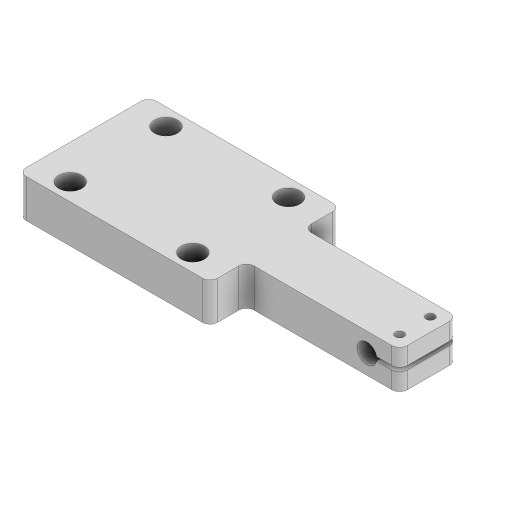
# Autodesk Inventor part: Puller
Saved by Autodesk Inventor 2023 (Build 270158000, 158)
## iProperties
Created: 2026-05-19
Part Number: Puller
Material: Generic
Document SubType Name: Modeling
Designer: ferrerx
Density: 1 g/cm^3
Appearance: Default
Author: ferrerx
Autodesk Inventor part; units mm, degrees
ref_plane "YZ Plane" through (0, 0, 0) normal (1, 0, 0) x (0, 1, 0)
ref_plane "XZ Plane" through (0, 0, 0) normal (0, 1, 0) x (-1, 0, 0)
ref_plane "XY Plane" through (0, 0, 0) normal (0, 0, 1) x (1, 0, 0)
sketch "Sketch1" plane through (0, 0, 0) normal (0, 1, 0) x (-1, 0, 0)
  line L0 (-16, 12.5) -> (16, 12.5) construction
  line L1 (16, 12.5) -> (16, -12.5) construction
  line L2 (16, -12.5) -> (-16, -12.5) construction
  line L3 (-16, -12.5) -> (-16, 12.5) construction
  line L4 (-16, 12.5) -> (16, -12.5) construction
  line L5 (16, 12.5) -> (-16, -12.5) construction
  circle A0 centre (16, 12.5) radius 1.65
  circle A1 centre (16, -12.5) radius 1.65
  circle A2 centre (-16, -12.5) radius 1.65
  circle A3 centre (-16, 12.5) radius 1.65
  line L6 (-25, 17) -> (25, 17)
  line L7 (25, 17) -> (25, -17)
  line L8 (25, -17) -> (-25, -17)
  line L9 (-25, -17) -> (-25, 17)
  line L10 (-25, 17) -> (25, -17) construction
  line L11 (25, 17) -> (-25, -17) construction
  point P0 (0, 0)
  dimension "d0" = 32
  dimension "d1" = 25
  dimension "d2" = 3.3
  dimension "d3" = 3.3
  dimension "d4" = 3.3
  dimension "d5" = 3.3
  dimension "d6" = 50
  dimension "d7" = 34
  constraints: 24 end point, 4 centre point, 4 coincident, 4 midpoint, 4 parallel, 2 horizontal, 2 perpendicular
  measures "d0" distance of L1.end L2.end
  measures "d1" distance of L0.end L1.end
  measures "d2" diameter of A0
  measures "d3" diameter of A1
  measures "d4" diameter of A2
  measures "d5" diameter of A3
  measures "d6" distance of L7.end L8.end
  measures "d7" distance of L6.end L7.end
extrude "Extrusion1" add sketch "Sketch1" along normal blind 10
sketch "Sketch2" plane through (0, 10, 0) normal (0, 1, 0) x (1, 0, 0)
  line L0 (-24, -7.5) -> (-12, -7.5)
  line L1 (-12, -7.5) -> (-12, 7.5)
  line L2 (-12, 7.5) -> (-24, 7.5)
  line L3 (-24, 7.5) -> (-24, -7.5)
  line L4 (-24, -7.5) -> (-12, 7.5) construction
  line L5 (-12, -7.5) -> (-24, 7.5) construction
  circle A0 centre (-16, -12.5) radius 1.65 projected
  circle A1 centre (-16, -12.5) radius 3 construction
  point P0 (0, 0)
  point P1 (-18, 0)
  dimension "d10" = 18
  dimension "d11" = 15
  dimension "d12" = 6
  dimension "d13" = 12
  constraints: 12 end point, 2 midpoint, 2 parallel, 1 centre point, 1 coincident, 1 horizontal, 1 perpendicular
  measures "d10" distance of point (0, 0) point (-18, 0)
  measures "d11" distance of L2.end L0.start
  measures "d12" diameter of A1
  measures "d13" distance of L1.end L2.end
extrude "Extrusion2" [suppressed]
sketch "Sketch5" plane through (0, 0, 0) normal (0, 0, 1) x (1, 0, 0)
  line L0 (25, 10) -> (-25, 10) projected
  line L1 (-21.2587, 10) -> (-11, 10)
  line L2 (-11, 10) -> (-11, 19.7515)
  line L3 (-11, 19.7515) -> (-17.6064, 31.6553)
  line L4 (-17.6064, 31.6553) -> (-28.0988, 25.8321)
  line L5 (-28.0988, 25.8321) -> (-21.2587, 13.5072)
  line L6 (-21.2587, 13.5072) -> (-21.2587, 10)
  circle A0 centre (-18, 20) radius 2.6308
  line L7 (-25, 0) -> (-25, 10) projected
  point P0 (0, 0)
  dimension "d22" = 7
  dimension "d23" = 10
  dimension "d24" = 7
  dimension "d26" = 6
  dimension "d27" = 6
  dimension "d28" = 10
  constraints: 13 end point, 2 perpendicular, 2 point on line, 1 centre point, 1 parallel, 1 vertical
  measures "d22" distance from line of L7 A0.centre
  measures "d23" distance from line of L0 A0.centre
  measures "d24" distance from line of A0.centre L2
  measures "d26" distance from line of L5 A0.centre
  measures "d27" distance from line of L3 A0.centre
  measures "d28" distance from line of A0.centre L4
extrude "Extrusion4" [suppressed]
sketch "Sketch6" plane through (-17.6064, 27.6553, 6) normal (0.8744, 0.4853, 0) x (0, 0, -1)
  circle A0 centre (3, -3) radius 1.1
  line L0 (12, 0) -> (0, 0) projected
  line L1 (0, -13.6141) -> (0, 0) projected
  line L2 (6, 0) -> (6, -13.6141) construction
  line L3 (12, -13.6141) -> (0, -13.6141) projected
  circle A1 centre (9, -3) radius 1.1
  point P0 (6, -32.7246)
  dimension "d31" = 3
  dimension "d32" = 3
  dimension "d38" = 2.2
  constraints: 2 centre point, 2 end point, 2 midpoint, 1 symmetric about line, 1 other
  measures "d31" distance from line of L0 A0.centre
  measures "d32" distance from line of L1 A0.centre
  measures "d38" diameter of A0
extrude "Extrusion5" [suppressed]
sketch "Sketch7" plane through (0, 0, 6) normal (0, 0, 1) x (1, 0, 0)
  line L0 (-28.2228, 33.3896) -> (-18.3568, 15.6125)
  line L1 (-18.3568, 15.6125) -> (-17.4824, 16.0978)
  line L2 (-17.4824, 16.0978) -> (-27.3485, 33.8749)
  line L3 (-27.3485, 33.8749) -> (-28.2228, 33.3896)
  line L4 (-17.6064, 27.6553) -> (-28.0988, 21.8321) projected
  line L5 (-28.2228, 33.3896) -> (-17.4824, 16.0978) construction
  line L6 (-18.3568, 15.6125) -> (-27.3485, 33.8749) construction
  point P0 (0, 0)
  point P1 (-22.8526, 24.7437)
  dimension "d35" = 1
  constraints: 12 end point, 3 midpoint, 2 parallel, 2 perpendicular
  measures "d35" distance between parallel lines of L2 L0
extrude "Extrusion6" [suppressed]
sketch "Sketch8" plane through (-21.2587, 9.5072, -6) normal (-0.8744, -0.4853, 0) x (0, 0, 1)
  circle A0 centre (9, 11.0958) radius 1.1 projected
  circle A1 centre (9, 11.0958) radius 1.65
  circle A2 centre (3, 11.0958) radius 1.1 projected
  circle A3 centre (3, 11.0958) radius 1.65
  point P0 (6, -18.6288)
  dimension "d39" = 3.3
  dimension "d40" = 3.3
  constraints: 2 centre point, 2 coincident
  measures "d39" diameter of A3
  measures "d40" diameter of A1
extrude "Extrusion7" [suppressed]
fillet "Fillet1" [suppressed]
chamfer "Chamfer1" [suppressed]
sketch "Sketch9" plane through (0, 10, 0) normal (0, 1, 0) x (1, 0, 0)
  circle A0 centre (-16, 12.5) radius 1.65 projected
  circle A1 centre (-16, 12.5) radius 3
  circle A2 centre (16, 12.5) radius 1.65 projected
  circle A3 centre (16, 12.5) radius 3
  circle A4 centre (16, -12.5) radius 1.65 projected
  circle A5 centre (16, -12.5) radius 3
  circle A6 centre (-16, -12.5) radius 1.65 projected
  circle A7 centre (-16, -12.5) radius 3
  point P0 (0, 0)
  dimension "d47" = 6
  dimension "d48" = 6
  dimension "d49" = 6
  dimension "d50" = 6
  constraints: 4 centre point, 4 coincident
  measures "d47" diameter of A1
  measures "d48" diameter of A3
  measures "d49" diameter of A5
  measures "d50" diameter of A7
extrude "Extrusion8" cut sketch "Sketch9" against normal blind 4 contours A0 | A1 | A3 | A5 | A7
fillet "Fillet2" radius 2 4 edges at (25, 5, 17) (25, 5, -17) (-25, 5, 17) (-25, 5, -17)
sketch "Sketch11" plane through (0, 0, 0) normal (0, 0, 1) x (1, 0, 0)
  line L0 (25, 10) -> (-25, 10) projected
  line L1 (25, 10) -> (65, 10)
  line L2 (65, 10) -> (65, 0)
  line L3 (65, 0) -> (25, 0)
  line L4 (25, 0) -> (25, 10)
  point P0 (0, 0)
  dimension "d54" = 40
  dimension "d55" = 10
  constraints: 8 end point, 2 parallel, 1 horizontal, 1 perpendicular
  measures "d54" distance of L0.start L1.end
  measures "d55" distance of L1.end L2.end
extrude "Extrusion9" add sketch "Sketch11" along normal mid plane 15
sketch "Sketch12" plane through (0, 0, -7.5) normal (0, 0, -1) x (-1, 0, 0)
  line L0 (-65, 10) -> (-65, 0) projected
  line L1 (-65, 5) -> (-56.5, 5) construction
  circle A0 centre (-56.5, 5) radius 2.55
  line L2 (-67.1062, 5.5) -> (-57.7546, 5.5)
  line L3 (-57.7546, 5.5) -> (-57.7546, 4.5)
  line L4 (-57.7546, 4.5) -> (-67.1062, 4.5)
  line L5 (-67.1062, 4.5) -> (-67.1062, 5.5)
  line L6 (-67.1062, 5.5) -> (-57.7546, 4.5) construction
  line L7 (-57.7546, 5.5) -> (-67.1062, 4.5) construction
  point P0 (0, 0)
  point P1 (-62.4304, 5)
  point P2 (-59.0005, 4.5)
  point P3 (-59.0005, 5.5)
  dimension "d58" = 5.1
  dimension "d59" = 8.5
  dimension "d67" = 1
  constraints: 14 end point, 3 midpoint, 2 horizontal, 2 parallel, 1 centre point, 1 coincident, 1 perpendicular, 1 point on line
  measures "d58" diameter of A0
  measures "d59" distance of L1.start L1.end
  measures "d67" distance between parallel lines of L2 L4
extrude "Extrusion10" cut sketch "Sketch12" against normal blind 15
sketch "Sketch13" plane through (0, 10, 0) normal (0, 1, 0) x (1, 0, 0)
  circle A0 centre (61.5, 4) radius 1.1
  line L0 (25, 7.5) -> (65, 7.5) projected
  line L1 (65, 7.5) -> (65, -7.5) projected
  line L2 (65, 7.5) -> (65, -7.5) projected
  line L3 (65, 0) -> (0, 0) construction
  circle A1 centre (61.5, -4) radius 1.1
  dimension "d62" = 3.5
  dimension "d63" = 3.5
  dimension "d64" = 2.2
  constraints: 2 centre point, 2 end point, 1 horizontal, 1 midpoint, 1 symmetric about line, 1 other
  measures "d62" distance from line of L0 A0.centre
  measures "d63" distance from line of A0.centre L1
  measures "d64" diameter of A0
extrude "Extrusion11" cut sketch "Sketch13" against normal blind 10.25
sketch "Sketch14" plane through (25, 0, 7.5) normal (0, -1, 0) x (1, 0, 0)
  circle A0 centre (36.5, -3.5) radius 1.1 projected
  circle A1 centre (36.5, -3.5) radius 1.6
  circle A2 centre (36.5, -11.5) radius 1.1 projected
  circle A3 centre (36.5, -11.5) radius 1.6
  point P0 (-25, -7.5)
  dimension "d68" = 3.2
  dimension "d69" = 3.2
  constraints: 2 centre point, 2 coincident
  measures "d68" diameter of A1
  measures "d69" diameter of A3
extrude "Extrusion12" cut sketch "Sketch14" against normal blind 4 contours A0 | A1 | A2 | A3
fillet "Fillet3" radius 2 4 edges at (65, 7.75, -7.5) (65, 2.25, -7.5) (65, 2.25, 7.5) (65, 7.75, 7.5)
fillet "Fillet4" radius 2 2 edges at (25, 5, -7.5) (25, 5, 7.5)
equation "\"d3\" = d2"
equation "\"d4\" = d2"
equation "\"d5\" = d2"
equation "\"d48\" = d47"
equation "\"d49\" = d47"
equation "\"d50\" = d47"
equation "\"d69\" = d68"
body "Solid1"
